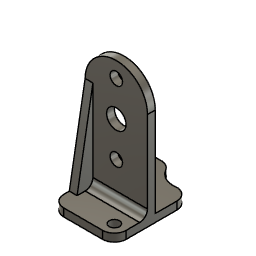
BLTouch Mount (Autodesk Fusion 360 design; units mm, degrees)
Autodesk Fusion 360 part; units mm, degrees
sketch "Sketch1" plane through (0, 0, 0) normal (0, 1, 0) x (1, 0, 0)
  line L0 (-4.9858, 11.5) -> (-2.9364, 11.5)
  line L1 (8, 4.5467) -> (8, -8.4858)
  line L2 (4.9858, -11.5) -> (-4.9858, -11.5)
  line L3 (-8, -8.4858) -> (-8, 8.4858)
  line L4 (-8, 11.5) -> (8, -11.5) construction
  line L5 (8, 11.5) -> (-8, -11.5) construction
  circle A0 centre (-5.0352, 8.5) radius 1.325
  arc A1 (-0.3276, 9.9956) -> (4.6151, 7.538) centre (4, 12.5) ccw
  arc A2 (-4.9858, 11.5) -> (-8, 8.4858) centre (-4.9858, 8.4858) ccw
  arc A3 (-0.3276, 9.9956) -> (-2.9364, 11.5) centre (-2.9364, 8.4858) ccw
  arc A4 (8, 4.5467) -> (4.6151, 7.538) centre (4.9858, 4.5467) ccw
  arc A5 (4.9858, -11.5) -> (8, -8.4858) centre (4.9858, -8.4858) ccw
  arc A6 (-8, -8.4858) -> (-4.9858, -11.5) centre (-4.9858, -8.4858) ccw
  circle A7 centre (5, -8.5) radius 1.325
  dimension "d74" = 10
  dimension "d75" = 12
  dimension "d76" = 2.65
  dimension "d77" = 3
  dimension "d79" = 4
  dimension "d81" = 2.65
  dimension "d82" = 3
  dimension "d83" = 3
  dimension "d84" = 16
  dimension "d85" = 23
  constraint horizontal L0
  constraint perpendicular L0 L1
  constraint parallel L0 L2
  constraint parallel L1 L3
  constraint coincident L4 origin
  constraint coincident L5 origin
  constraint coincident L4.start L0
  constraint coincident L4.start L3
  constraint tangent L0 A2
  constraint tangent L3 A2
  constraint tangent L0 A3
  constraint tangent A1 A3
  constraint equal A2 A3
  constraint tangent A1 A4
  constraint tangent L1 A4
  constraint equal A2 A4
  constraint coincident L4.end L1
  constraint coincident L4.end L2
  constraint tangent L1 A5
  constraint tangent L2 A5
  constraint equal A2 A5
  constraint coincident L5.end L2
  constraint coincident L5.end L3
  constraint tangent L2 A6
  constraint tangent L3 A6
  constraint equal A2 A6
  constraint coincident L5.start L1
  constraint coincident L5.start L0
  measures "d74" diameter of A1
  measures "d75" distance of L3 A1.centre
  measures "d76" diameter of A0
  measures "d77" distance of L0 A0.centre
  measures "d79" vertical distance of A1.centre A0.centre
  measures "d81" diameter of A7
  measures "d82" distance of L1 A7.centre
  measures "d83" distance of L2 A7.centre
  measures "d84" distance of L1 L3
  measures "d85" distance of L0 L2
extrude "Extrude1" add sketch "Sketch1" against normal blind 2
ref_plane "WorkPlane1" through (0, 0, 2) normal (0, 0, 1) x (1, 0, 0)
sketch "Sketch14" plane through (0, 0, 2) normal (0, 0, 1) x (1, 0, 0)
  line L0 (-8, 0) -> (8, 0)
  circle A0 centre (0, 18) radius 2.5
  circle A1 centre (0, 27) radius 1.6
  arc A2 (8, 23) -> (0, 31) centre (0, 23) ccw
  line L1 (-8, 23) -> (-8, 0)
  arc A3 (0, 31) -> (-8, 23) centre (0, 23) ccw
  line L2 (8, 0) -> (8, 23)
  circle A4 centre (0, 9) radius 1.6
  point P0 (-8, 31)
  dimension "d64" = 16
  dimension "d65" = 31
  dimension "d66" = 3.2
  dimension "d67" = 3.2
  dimension "d68" = 18
  dimension "d69" = 5
  dimension "d70" = 9
  dimension "d71" = 8
  constraint horizontal L0
  constraint vertical L2
  constraint vertical L1
  constraint vertical A4.centre A1.centre
  constraint vertical origin A0.centre
  constraint vertical origin A4.centre
  constraint midpoint origin L0
  constraint coincident P0 L1
  constraint tangent L1 A3
  constraint tangent A2 L2
  constraint equal A2 A3
  constraint coincident A2.end A3.start
  measures "d64" distance of L0.end L0.start
  measures "d65" distance of L0.start P0
  measures "d66" diameter of A1
  measures "d67" diameter of A4
  measures "d68" vertical distance of A4.centre A1.centre
  measures "d69" diameter of A0
  measures "d70" vertical distance of A0.centre A1.centre
  measures "d71" radius of A3
extrude "Extrude8" add sketch "Sketch14" along normal mid plane 2
sketch "Sketch16" plane through (-8, 0, 0) normal (-1, 0, 0) x (0, 0, 1)
  line L0 (8.4858, 0) -> (3, 0)
  line L1 (3, 0) -> (3, 23)
  line L2 (3, 23) -> (1, 23)
  line L3 (1, 23) -> (1, 0)
  line L4 (1, 0) -> (-8.4858, 0)
  line L5 (-8.4858, 0) -> (-8.4858, -2)
  line L6 (-8.4858, -2) -> (8.4858, -2)
  line L7 (8.4858, -2) -> (8.4858, 0)
  line L8 (3, 23) -> (7.0555, 0)
  line L9 (3, 23) -> (26.3548, 23) construction
  dimension "d86" = 80
  constraint horizontal L9
  constraint coincident L1.end L2.start
  constraint coincident L0 L8.end
  measures "d86" angle of L8 L9
extrude "Extrude9" add sketch "Sketch16" against normal blind 2 contours L0 L1 L8
fillet "Fillet3" radius 2 1 edges at (1, 0, 3)
equation "d65 = 26 mm + 5 mm"
equation "d71 = ( 16 / 2 ) * 1 mm"
equation "d72 = ( 2 / 2 ) * 1 mm"
